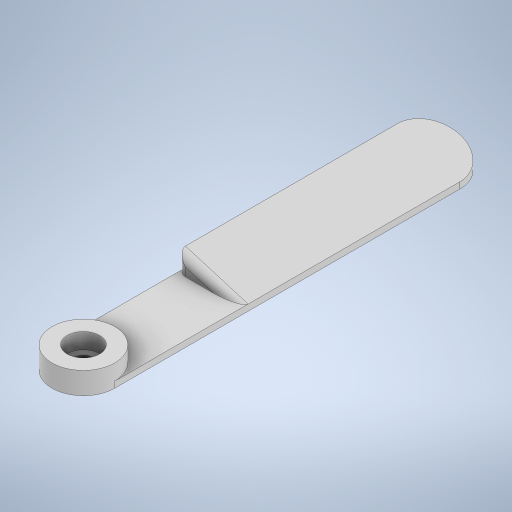
# Autodesk Inventor part: Pbj5
Saved by Autodesk Inventor 2023.1 (Build 271208000, 208)
## iProperties
Created: 2023-04-24
Part Number: Pbj5
Material: Generisch
Document SubType Name: Sheet Metal
Designer: marco
Density: 1 g/cm^3
Sheet Metal Rule: Standard_mm
Appearance: Vorgabe
Author: marco
Autodesk Inventor part; units mm, degrees
ref_plane "YZ Plane" through (0, 0, 0) normal (1, 0, 0) x (0, 1, 0)
ref_plane "XZ Plane" through (0, 0, 0) normal (0, 1, 0) x (-1, 0, 0)
ref_plane "XY Plane" through (0, 0, 0) normal (0, 0, 1) x (1, 0, 0)
sketch "Skizze1" plane through (0, 0, 0) normal (0, 1, 0) x (-1, 0, 0)
  circle A0 centre (0, 0) radius 2.6
  circle A1 centre (0, 0) radius 5
  line L0 (5, 0) -> (-5, 0)
  line L1 (-5, 0) -> (-5, -60)
  line L2 (-5, -60) -> (5, -60)
  line L3 (5, -60) -> (5, 0)
  circle A2 centre (0, -55) radius 5
  point P0 (-5, -55)
  point P1 (5, -55)
  dimension "d1" = 10
  dimension "d0" = 5.2
  dimension "d2" = 60
  constraints: 8 end point, 2 centre point, 2 coincident, 2 parallel, 1 horizontal, 1 perpendicular, 3 other
  measures "d0" diameter of A0
  measures "d2" distance of L1.end L0.end
extrude "Extrusion1" add sketch "Skizze1" along normal blind 1 contours L0 A0 | L0 A1 A0 | A0 L0 A1 | A0 L0 | L3 A2 L1 A1 | A2
sketch "Skizze2" plane through (0, 1, 0) normal (0, 1, 0) x (1, 0, 0)
  circle A0 centre (0, 0) radius 2.575
  line L0 (-5, 55) -> (-5, 0) projected
  circle A1 centre (0, 0) radius 5
  dimension "d5" = 5.15
  constraints: 2 coincident, 1 centre point, 1 horizontal alignment, 2 other
  measures "d5" diameter of A0
extrude "Extrusion2" add sketch "Skizze2" along normal blind 2.5
sketch "Skizze3" plane through (0, 1, 0) normal (0, 1, 0) x (1, 0, 0)
  circle A0 centre (0, 0) radius 1.5
  dimension "d8" = 3
  constraints: 1 centre point, 1 coincident
  measures "d8" diameter of A0
extrude "Extrusion3" cut sketch "Skizze3" against normal blind 2.5
sketch "Skizze5" plane through (0, 1, 0) normal (0, 1, 0) x (1, 0, 0)
  arc A0 (5, 55) -> (-5, 55) centre (0, 55) ccw projected
  line L0 (5, 20) -> (-5, 20)
  line L1 (-5, 20) -> (-5, 55)
  line L2 (-5, 55) -> (5, 55)
  line L3 (5, 55) -> (5, 20)
  arc A1 (5, 55) -> (-5, 55) centre (0, 55) ccw
  point P0 (0, 0)
  constraints: 8 end point, 2 parallel, 2 point on circle, 2 tangent, 1 centre point, 1 horizontal, 1 perpendicular
extrude "Extrusion4" add sketch "Skizze5" along normal blind 3
sketch "Skizze6" plane through (-5, 1, -20) normal (0, 0, 1) x (1, 0, 0)
  line L0 (0, 0) -> (0, 3) projected
  line L1 (0, 3) -> (0, 0)
  line L2 (10, 0) -> (0, 0) projected
  line L3 (0, 0) -> (10, 0)
  line L4 (0, 3) -> (10, 3) projected
  line L5 (10, 0) -> (0, 3)
  line L6 (0, -1) -> (0, 3) projected
  line L7 (0, 3) -> (10, 3)
  line L8 (10, -1) -> (10, 3) projected
  line L9 (10, 3) -> (10, 0)
  point P0 (5, -1)
  constraints: 10 end point, 3 collinear, 1 horizontal
extrude "Extrusion5" cut sketch "Skizze6" against normal blind 47 contours L4 L8 L5
fillet "Rundung1" radius 1.25 2 edges at (0, 2.5, -20) (-5, 2.5, -20)
equation "\"Biegeradius\" = Stärke"
equation "\"BreiteBiegungsfreistellung\" = Stärke"
equation "\"TiefeBiegungsfreistellung\" = 0.5 * Stärke"
equation "\"GrößeEckenfreistellung\" = 4 * Stärke"
equation "\"MinimalRest\" = 2 * Stärke"
equation "\"Übergangsradius\" = Biegeradius"
equation "\"JacobiRadiusGröße\" = Biegeradius"
equation "\"Abstandsgröße\" = Stärke"
equation "\"Stärke\" = 0.5"
